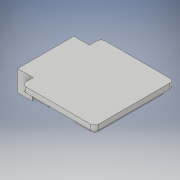
# Autodesk Inventor part: Enclosure_Top V2D6
Saved by Autodesk Inventor 2017 (Build 210142000, 142)
## iProperties
Created: 2018-02-12
Part Number: Enclosure_Top V2D6
Material: Generic
Document SubType Name: Modeling
Designer: Tripl_000
Density: 1 g/cm^3
Appearance: Default
Author: Tripl_000
Autodesk Inventor part; units mm, degrees
ref_plane "YZ Plane" through (0, 0, 0) normal (1, 0, 0) x (0, 1, 0)
ref_plane "XZ Plane" through (0, 0, 0) normal (0, 1, 0) x (-1, 0, 0)
ref_plane "XY Plane" through (0, 0, 0) normal (0, 0, 1) x (1, 0, 0)
sketch "Sketch1" plane through (0, 0, 0) normal (0, 1, 0) x (-1, 0, 0)
  line L0 (15.5, 17.05) -> (-15.5, 17.05)
  line L1 (-15.5, 17.05) -> (-15.5, -17.05)
  line L2 (-15.5, -17.05) -> (15.5, -17.05)
  line L3 (15.5, -17.05) -> (15.5, 17.05)
  line L4 (15.5, 17.05) -> (-15.5, -17.05) construction
  line L5 (-15.5, 17.05) -> (15.5, -17.05) construction
  point P0 (0, 0)
  dimension "d0" = 31
  dimension "d1" = 34.1
  constraints: 12 end point, 2 midpoint, 2 parallel, 1 horizontal, 1 perpendicular
  measures "d0" distance between parallel lines of L1 L3
  measures "d1" distance between parallel lines of L0 L2
extrude "Extrusion1" add sketch "Sketch1" along normal blind 2.5
sketch "Sketch2" plane through (0, 2.5, 0) normal (0, 1, 0) x (1, 0, 0)
  line L0 (-17.5, -19.05) -> (17.5, -19.05)
  line L1 (17.5, -19.05) -> (17.5, 19.05)
  line L2 (17.5, 19.05) -> (-17.5, 19.05)
  line L3 (-17.5, 19.05) -> (-17.5, -19.05)
  line L4 (-17.5, -19.05) -> (17.5, 19.05) construction
  line L5 (17.5, -19.05) -> (-17.5, 19.05) construction
  point P0 (0, 0)
  dimension "d4" = 35
  dimension "d5" = 38.1
  constraints: 12 end point, 2 midpoint, 2 parallel, 1 horizontal, 1 perpendicular
  measures "d4" distance between parallel lines of L1 L3
  measures "d5" distance between parallel lines of L0 L2
extrude "Extrusion2" add sketch "Sketch2" along normal blind 2.5
sketch "Sketch3" plane through (0, 0, 0) normal (0, -1, 0) x (1, 0, 0)
  line L0 (-15.5, 17.05) -> (15.5, 17.05) projected
  line L1 (0, 17.05) -> (6.5, 17.05)
  line L2 (6.5, 17.05) -> (6.5, -26.1554)
  line L3 (6.5, -26.1554) -> (0, -26.1554)
  line L4 (0, -26.1554) -> (0, 17.05)
  point P0 (0, 0)
  dimension "d8" = 6.5
  constraints: 8 end point, 2 parallel, 1 horizontal, 1 midpoint, 1 perpendicular
  measures "d8" distance between parallel lines of L4 L2
extrude "Extrusion3" cut sketch "Sketch3" against normal up to surface (2.5 mm away)
ref_plane "Work Plane1" through (0, 0, 17.05) normal (1, 0, 0) x (0, 0, -1)
mirror "Mirror1" about plane through (0, 0, 17.05) normal (1, 0, 0) of "Extrusion3"
sketch "Sketch4" plane through (0, 0, 0) normal (0, -1, 0) x (1, 0, 0)
  line L0 (-6.5, -17.05) -> (-6.5, 17.05) projected
  line L1 (-15.5, -17.05) -> (-15.5, 17.05) projected
  line L2 (-6.5, 0) -> (-15.5, 0)
  line L3 (-15.5, 0) -> (-15.5, 11)
  line L4 (-15.5, 11) -> (-6.5, 11)
  line L5 (-6.5, 11) -> (-6.5, 0)
  point P0 (0, 0)
  dimension "d12" = 11
  constraints: 8 end point, 2 parallel, 1 horizontal, 1 midpoint, 1 perpendicular, 1 point on line
  measures "d12" distance between parallel lines of L4 L2
extrude "Extrusion4" cut sketch "Sketch4" against normal blind 4
ref_plane "Work Plane2" through (-15.5, 0, 0) normal (0, 0, 1) x (1, 0, 0)
sketch "Sketch5" plane through (-17.5, 2.5, -19.05) normal (-1, 0, 0) x (0, 0, 1)
  line L0 (2, 0) -> (36.1, 0) projected
  line L1 (0, 2.5) -> (38.1, 2.5) projected
  line L2 (30.05, 0) -> (19.05, 0)
  line L3 (19.05, 0) -> (19.05, 2.5)
  line L4 (19.05, 2.5) -> (30.05, 2.5)
  line L5 (30.05, 2.5) -> (30.05, 0)
  point P0 (19.05, -2.5)
  dimension "d16" = 11
  constraints: 8 end point, 2 parallel, 1 horizontal, 1 midpoint, 1 perpendicular, 1 point on line
  measures "d16" distance between parallel lines of L5 L3
extrude "Extrusion5" add sketch "Sketch5" along normal blind 7.5
sketch "Sketch6" plane through (-17.5, 2.5, 11) normal (0, 0, 1) x (1, 0, 0)
  line L0 (0, 2.5) -> (0, 0) projected
  line L1 (-7.5, 0) -> (0, 0)
  line L2 (0, 0) -> (0, 2.5)
  line L3 (0, 2.5) -> (-7.5, 2.5)
  line L4 (-7.5, 2.5) -> (-7.5, 0)
  point P0 (17.5, -2.5)
  constraints: 8 end point, 2 parallel, 1 horizontal, 1 perpendicular
extrude "Extrusion6" add sketch "Sketch6" along normal blind 2.5
sketch "Sketch7" plane through (0, 2.5, 0) normal (0, -1, 0) x (1, 0, 0)
  line L0 (-25, 0) -> (-25, 13.5) projected
  line L1 (-25, 13.5) -> (-18, 13.5)
  line L2 (-18, 13.5) -> (-18, 11)
  line L3 (-18, 11) -> (-22.5, 11)
  line L4 (-25, 11) -> (-25, 13.5)
  line L5 (-15.5, 11) -> (-15.5, 17.05) projected
  line L6 (-17.5, 0) -> (-25, 0) projected
  line L7 (-22.5, 11) -> (-22.5, 0)
  line L8 (-22.5, 0) -> (-25, 0)
  line L9 (-25, 0) -> (-25, 11)
  point P0 (0, 0)
  dimension "d21" = 2.5
  dimension "d23" = 2.5
  dimension "d24" = 7
  constraints: 14 end point, 3 parallel, 1 horizontal, 1 perpendicular, 1 point on line
  measures "d21" distance between parallel lines of L3 L1
  measures "d23" distance between parallel lines of L0 L7
  measures "d24" distance of L0.end L1.end
extrude "Extrusion7" add sketch "Sketch7" along normal blind 7.5
mirror "Mirror2" about plane through (-15.5, 0, 0) normal (0, 0, 1) of "Extrusion4", "Extrusion5", "Extrusion6", "Extrusion7"
fillet "Fillet1" radius 2 8 edges at (17.5, 3.75, 19.05) (15.5, 1.25, 17.05) (17.5, 3.75, -19.05) (15.5, 1.25, -17.05) (-17.5, 3.75, -19.05) (-15.5, 1.25, -17.05) (-17.5, 3.75, 19.05) (-15.5, 1.25, 17.05)
fillet "Fillet2" radius 5 1 edges at (-22.5, 2.5, 0)
body "Solid1"
